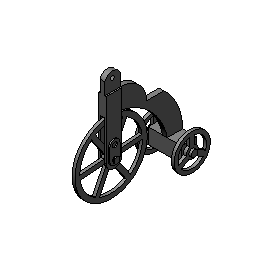
Monkey_Riding_Bike v2 (Autodesk Fusion 360 design; units mm, degrees)
Autodesk Fusion 360 part; units mm, degrees
sketch "Wheels holder" plane through (0, 0, 0) normal (1, 0, 0) x (0, 1, 0) in component "Bike"
  line L0 (89.0864, -65.3231) -> (57.0864, -65.3231)
  line L1 (57.0864, -65.3231) -> (57.0864, -97.3231)
  line L2 (57.0864, -97.3231) -> (89.0864, -97.3231)
  line L3 (89.0864, -97.3231) -> (89.0864, -65.3231)
  line L4 (89.0864, -65.3231) -> (57.0864, -97.3231) construction
  line L5 (57.0864, -65.3231) -> (89.0864, -97.3231) construction
  point P0 (73.0864, -81.3231)
  dimension "d1" = 32
  dimension "d2" = 32
  constraint horizontal L0
  constraint perpendicular L0 L1
  constraint parallel L0 L2
  constraint parallel L1 L3
  constraint coincident L4 P0
  constraint coincident L5 P0
  measures "d1" distance of L1.end L2.end
  measures "d2" distance of L0.end L1.end
extrude "Extrude1" add sketch "Wheels holder" along normal mid plane 69 makes body 1 in component "Bike"
sketch "Bike" plane through (0, 0, 0) normal (1, 0, 0) x (0, 1, 0) in component "Bike"
  line L0 (50.0158, 22.6931) -> (15, 22.6931)
  line L1 (-40, 75) -> (-40, 100)
  line L2 (-72.5145, 100) -> (-72.5145, 35)
  line L3 (57.3009, -65.5095) -> (89.0864, -65.3233)
  arc A0 (57.3009, -65.5095) -> (-72.5145, 35) centre (-65.2547, -89.7112) ccw
  arc A1 (89.0864, -65.3233) -> (50.0158, 22.6931) centre (-30.4896, -65.7234) ccw
  arc A2 (15, 22.6931) -> (-40, 75) centre (-39.9292, 20.0051) ccw
  arc A3 (-40, 100) -> (-72.5145, 100) centre (-56.2572, 94.6148) ccw
  constraint horizontal L0
  constraint vertical L1
extrude "Extrude2" add sketch "Bike" along normal mid plane 10 bodies 1 in component "Bike"
sketch "Wheel" plane through (0, 0, 0) normal (1, 0, 0) x (0, 1, 0) in component "Big wheel"
  circle A0 centre (-57.5, -44) radius 75
  line L0 (-57.6215, -58.9995) -> (-40.7303, -106.7995)
  line L1 (-48.5271, -56.0203) -> (-31.6934, -103.6575)
  line L2 (-44.5708, -51.605) -> (5.2708, -60.8767)
  line L3 (-42.6037, -42.2394) -> (7.0682, -51.4796)
  line L4 (-44.4493, -36.6055) -> (-11.4989, 1.9228)
  line L5 (-51.5765, -30.2191) -> (-18.7384, 8.1779)
  line L6 (-57.3785, -29.0005) -> (-74.2697, 18.7995)
  line L7 (-66.4729, -31.9797) -> (-83.3066, 15.6575)
  line L8 (-70.4292, -36.395) -> (-120.2708, -27.1233)
  line L9 (-72.3963, -45.7606) -> (-122.0682, -36.5204)
  line L10 (-70.5507, -51.3945) -> (-103.5011, -89.9228)
  line L11 (-63.4235, -57.7809) -> (-96.2616, -96.1779)
  arc A1 (-18.7384, 8.1779) -> (-74.2697, 18.7995) centre (-57.5, -44) ccw
  arc A2 (-51.5765, -30.2191) -> (-57.3785, -29.0005) centre (-57.5, -44) ccw
  arc A3 (-42.6037, -42.2394) -> (-44.4493, -36.6055) centre (-57.5, -44) ccw
  arc A4 (7.0682, -51.4796) -> (-11.4989, 1.9228) centre (-57.5, -44) ccw
  arc A5 (-48.5271, -56.0203) -> (-44.5708, -51.605) centre (-57.5, -44) ccw
  arc A6 (-63.4235, -57.7809) -> (-57.6215, -58.9995) centre (-57.5, -44) ccw
  arc A7 (-66.4729, -31.9797) -> (-70.4292, -36.395) centre (-57.5, -44) ccw
  arc A8 (-72.3963, -45.7606) -> (-70.5507, -51.3945) centre (-57.5, -44) ccw
  arc A9 (-83.3066, 15.6575) -> (-120.2708, -27.1233) centre (-57.5, -44) ccw
  arc A10 (-122.0682, -36.5204) -> (-103.5011, -89.9228) centre (-57.5, -44) ccw
  arc A11 (-96.2616, -96.1779) -> (-40.7303, -106.7995) centre (-57.5, -44) ccw
  arc A12 (-31.6934, -103.6575) -> (5.2708, -60.8767) centre (-57.5, -44) ccw
  dimension "d7" = 150
  dimension "d9" = 30
  dimension "d11" = 360
  constraint concentric A0 A7
  constraint coincident L0.end A9
  constraint coincident L1.start A7
  constraint coincident L1.end A9
  constraint parallel L0 L1
  constraint concentric A0 A9
  constraint concentric A1 A9
  constraint concentric A2 A7
  constraint concentric A3 A7
  constraint concentric A4 A9
  constraint concentric A5 A7
  constraint concentric A6 A7
  constraint concentric A7 A8
  constraint concentric A9 A10
  constraint concentric A10 A11
  constraint concentric A11 A12
  measures "d7" diameter of A0
  measures "d9" diameter of A7
extrude "Extrude1'" add sketch "Wheel" along normal mid plane 6 separate body makes body 2 in component "Big wheel"
sketch "Wheel (2)" plane through (0, 0, 0) normal (1, 0, 0) x (0, 1, 0) in component "Small wheels"
  circle A0 centre (73.0864, -81.3232) radius 37.5
  line L0 (68.0057, -69.9023) -> (68.0057, -52.264)
  line L1 (78.1671, -69.9023) -> (78.1671, -52.264)
  line L2 (65.7359, -91.4336) -> (50.4607, -100.2528)
  line L3 (60.6552, -82.6336) -> (45.38, -91.4528)
  line L4 (85.5175, -82.6336) -> (100.7927, -91.4528)
  line L5 (80.4368, -91.4336) -> (95.712, -100.2528)
  arc A1 (68.0057, -52.264) -> (45.38, -91.4528) centre (73.0864, -81.3232) ccw
  arc A2 (68.0057, -69.9023) -> (60.6552, -82.6336) centre (73.0864, -81.3232) ccw
  arc A3 (65.7359, -91.4336) -> (80.4368, -91.4336) centre (73.0864, -81.3232) ccw
  arc A4 (85.5175, -82.6336) -> (78.1671, -69.9023) centre (73.0864, -81.3232) ccw
  arc A5 (50.4607, -100.2528) -> (95.712, -100.2528) centre (73.0864, -81.3232) ccw
  arc A6 (100.7927, -91.4528) -> (78.1671, -52.264) centre (73.0864, -81.3232) ccw
  dimension "d14" = 75
  dimension "d16" = 25
  dimension "d18" = 360
  constraint concentric A0 A3
  constraint coincident L0.start A3
  constraint vertical L0
  constraint parallel L0 L1
  constraint concentric A0 A1
  constraint concentric A1 A5
  constraint concentric A2 A3
  constraint concentric A3 A4
  constraint concentric A5 A6
  measures "d14" diameter of A0
  measures "d16" diameter of A3
extrude "Extrude1''" add sketch "Wheel (2)" along normal blind 41 and the other way blind -35 separate body makes body 3 in component "Small wheels"
extrude "Extrude2'" add sketch "Wheel (2)" along normal blind -35 and the other way blind 41 separate body makes body 4 in component "Small wheels"
sketch "Bike pedals and wheel holder" plane through (5, 0, 0) normal (1, 0, 0) x (0, 1, 0) in component "Bike"
  line L0 (57.264, -65.3231) -> (89.0864, -65.3231)
  arc A0 (89.0864, -65.3231) -> (50.0158, 22.6931) centre (-30.4896, -65.7234) ccw
  line L1 (50.0158, 22.6931) -> (15, 22.6931)
  arc A1 (15, 22.6931) -> (-40, 75) centre (-39.9292, 20.0051) ccw
  line L2 (-40, 75) -> (-40, 100)
  arc A2 (-40, 100) -> (-72.5145, 100) centre (-56.2572, 94.6148) ccw
  line L3 (-72.5145, 100) -> (-72.5145, 35)
  arc A3 (57.264, -65.3231) -> (-72.5145, 35) centre (-65.2547, -89.7112) ccw
  line L4 (-40, 75) -> (-72.5145, 75)
  line L5 (-72.5145, 75) -> (-72.5145, -46.3572)
  line L6 (-40, -46.3572) -> (-40, 75)
  arc A4 (-72.5145, -46.3572) -> (-40, -46.3572) centre (-56.2572, -46.3572) ccw
  constraint horizontal L4
  constraint vertical L5
  constraint vertical L6
  constraint coincident A1.end L2.start
  constraint tangent L5 A4
extrude "Extrude3" add sketch "Bike pedals and wheel holder" along normal blind 3 contours A3 L5 L6 A4 | L3 A3 L4 L5 L6 bodies 1 in component "Bike"
extrude "Extrude4" add sketch "Bike pedals and wheel holder" along normal blind -10 and the other way blind 13 contours A3 L5 L6 A4 | L3 A3 L4 L5 L6 bodies 1 in component "Bike"
sketch "Bike hole" plane through (5, 0, 0) normal (1, 0, 0) x (0, 1, 0) in component "Bike"
  circle A0 centre (-56.5863, 99.3164) radius 4
  dimension "d33" = 8
  measures "d33" diameter of A0
extrude "Extrude5" cut sketch "Bike hole" against normal blind 175 bodies 1 in component "Bike"
sketch "Wheel Hole" plane through (41, 0, 0) normal (1, 0, 0) x (0, 1, 0) in component "Small wheels"
  line L0 (100.7927, -91.4528) -> (85.5175, -82.6336)
  arc A0 (85.5175, -82.6336) -> (78.1671, -69.9023) centre (73.0864, -81.3232) ccw
  line L1 (78.1671, -69.9023) -> (78.1671, -52.264)
  arc A1 (100.7927, -91.4528) -> (78.1671, -52.264) centre (73.0864, -81.3232) ccw
  arc A2 (68.0057, -52.264) -> (45.38, -91.4528) centre (73.0864, -81.3232) ccw
  line L2 (68.0057, -52.264) -> (68.0057, -69.9023)
  arc A3 (68.0057, -69.9023) -> (60.6552, -82.6336) centre (73.0864, -81.3232) ccw
  line L3 (60.6552, -82.6336) -> (45.38, -91.4528)
  line L4 (50.4607, -100.2528) -> (65.7359, -91.4336)
  arc A4 (65.7359, -91.4336) -> (80.4368, -91.4336) centre (73.0864, -81.3232) ccw
  line L5 (80.4368, -91.4336) -> (95.712, -100.2528)
  arc A5 (50.4607, -100.2528) -> (95.712, -100.2528) centre (73.0864, -81.3232) ccw
  circle A6 centre (73.0864, -81.3232) radius 37.5
  circle A7 centre (73.0864, -81.3232) radius 3.9
  circle A8 centre (73.0864, -81.3232) radius 3.5
  dimension "d36" = 7.8
  dimension "d72" = -0.4
  constraint concentric A0 A7
  measures "d36" diameter of A7
sketch "Wheel hole" plane through (3, -1, 0) normal (1, 0, 0) x (0, 1, 0) in component "Big wheel"
  line L0 (-30.6934, -103.6575) -> (-47.5271, -56.0203)
  arc A0 (-47.5271, -56.0203) -> (-43.5708, -51.605) centre (-56.5, -44) ccw
  line L1 (-43.5708, -51.605) -> (6.2708, -60.8767)
  arc A1 (-30.6934, -103.6575) -> (6.2708, -60.8767) centre (-56.5, -44) ccw
  line L2 (8.0682, -51.4796) -> (-41.6037, -42.2394)
  arc A2 (-41.6037, -42.2394) -> (-43.4493, -36.6055) centre (-56.5, -44) ccw
  line L3 (-43.4493, -36.6055) -> (-10.4989, 1.9228)
  arc A3 (8.0682, -51.4796) -> (-10.4989, 1.9228) centre (-56.5, -44) ccw
  line L4 (-82.3066, 15.6575) -> (-65.4729, -31.9797)
  arc A4 (-65.4729, -31.9797) -> (-69.4292, -36.395) centre (-56.5, -44) ccw
  line L5 (-69.4292, -36.395) -> (-119.2708, -27.1233)
  arc A5 (-82.3066, 15.6575) -> (-119.2708, -27.1233) centre (-56.5, -44) ccw
  arc A6 (-17.7384, 8.1779) -> (-73.2697, 18.7995) centre (-56.5, -44) ccw
  line L6 (-17.7384, 8.1779) -> (-50.5765, -30.2191)
  arc A7 (-50.5765, -30.2191) -> (-56.3785, -29.0005) centre (-56.5, -44) ccw
  line L7 (-56.3785, -29.0005) -> (-73.2697, 18.7995)
  line L8 (-121.0682, -36.5204) -> (-71.3963, -45.7606)
  arc A8 (-71.3963, -45.7606) -> (-69.5507, -51.3945) centre (-56.5, -44) ccw
  line L9 (-69.5507, -51.3945) -> (-102.5011, -89.9228)
  arc A9 (-121.0682, -36.5204) -> (-102.5011, -89.9228) centre (-56.5, -44) ccw
  line L10 (-95.2616, -96.1779) -> (-62.4235, -57.7809)
  arc A10 (-62.4235, -57.7809) -> (-56.6215, -58.9995) centre (-56.5, -44) ccw
  line L11 (-56.6215, -58.9995) -> (-39.7303, -106.7995)
  arc A11 (-95.2616, -96.1779) -> (-39.7303, -106.7995) centre (-56.5, -44) ccw
  circle A12 centre (-56.5, -44) radius 75
  circle A13 centre (-56.5, -44) radius 5
  dimension "d47" = 10
  constraint concentric A0 A13
  measures "d47" diameter of A13
extrude "Extrude8" cut sketch "Wheel hole" along normal mid plane 40 contours A13 bodies 1 in component "Bike"
extrude "Extrude2''" cut sketch "Wheel hole" along normal mid plane 40 contours A13 bodies 2 in component "Big wheel"
sketch "Pedal" plane through (8, 0, 0) normal (1, 0, 0) x (0, 1, 0) in component "Pedals"
  circle A0 centre (-57.5, -44) radius 5
  arc A1 (-72.5145, -46.3572) -> (-40, -46.3572) centre (-56.2572, -46.3572) ccw
  line L0 (-40, -46.3572) -> (-40, 75)
  line L1 (-40, 75) -> (-72.5145, 75)
  line L2 (-72.5145, 75) -> (-72.5145, -46.3572)
  line L3 (-47, -44) -> (-47, -18)
  arc A2 (-47, -18) -> (-68, -18) centre (-57.5, -18) ccw
  line L4 (-68, -18) -> (-68, -44)
  arc A3 (-68, -44) -> (-47, -44) centre (-57.5, -44) ccw
  line L5 (-57.5, -44) -> (-57.5, -18) construction
  circle A4 centre (-57.5, -44) radius 5
  circle A5 centre (-57.5, -18) radius 5
  dimension "d52" = 10
  constraint tangent L3 A2
  constraint tangent A2 L4
  constraint parallel L3 L4
  constraint tangent L4 A3
  constraint tangent L3 A3
  constraint vertical L5
  constraint coincident A0.centre A3.centre
  constraint concentric A3 A4
  constraint concentric A2 A5
  measures "d52" diameter of A5
extrude "Extrude1'''" add sketch "Pedal" along normal blind 3 separate body contours L3 A2 L4 A3 makes body 5 in component "Pedals"
extrude "Extrude2'''" add sketch "Pedal" along normal blind -19 and the other way blind 16 separate body contours L3 A2 L4 A3 makes body 6 in component "Pedals"
extrude "Extrude9" cut sketch "Wheel Hole" against normal blind 85 contours A7 | A8 bodies 1 in component "Bike"
move_face "OffsetFaces1" offset -0.3 1 faces at (11.5, 76.967, -81.7115) on bodies 1 in component "Bike"
extrude "Extrude3'" add sketch "Pedal" along normal blind -21 and the other way blind -5 separate body contours A0 A4 makes body 7 in component "Pedals"
move_face "OffsetFaces1'" offset -0.3 1 faces at (4.3333, -52.5248, -44.4978) on bodies 7 in component "Pedals"
move_face "OffsetFaces2" offset -0.4 2 faces at (8, -65.7218, -27.8003) (-8, -65.7218, -27.8003) on bodies 5 6 in component "Pedals"
extrude "Extrude6" cut sketch "Wheel Hole" against normal blind 160 contours A7 | A8 bodies 3 4 in component "Small wheels"
extrude "Extrude7" add sketch "Wheel Hole" along normal blind -30 and the other way blind 0 separate body contours A8 makes body 8 in component "Small wheels"
extrude "Extrude8'" add sketch "Wheel Hole" along normal blind -51 and the other way blind 82 separate body contours A8 makes body 9 in component "Small wheels"
sketch "Wheel screw" plane through (41, 0, 0) normal (1, 0, 0) x (0, 1, 0) in component "Small wheels"
  circle A0 centre (73.0864, -81.3232) radius 3.5
  circle A1 centre (73.0864, -81.3232) radius 7
  dimension "d81" = 14
  constraint concentric A0 A1
  measures "d81" diameter of A1
extrude "Extrude9'" add sketch "Wheel screw" along normal blind 5 contours A0 | A1 bodies 8 in component "Small wheels"
extrude "Extrude10" add sketch "Wheel screw" along normal blind -82 and the other way blind 87 contours A0 | A1 bodies 9 in component "Small wheels"
sketch "Connecting rod" plane through (13, 0, 0) normal (1, 0, 0) x (0, 1, 0) in component "Pedals"
  circle A0 centre (-57.5, -44) radius 4.7
  circle A1 centre (-57.5, -44) radius 6
  dimension "d88" = 12
  constraint concentric A0 A1
  measures "d88" diameter of A1
extrude "Extrude4'" add sketch "Connecting rod" along normal blind 2 contours A0 | A1 bodies 7 in component "Pedals"
component "Bike" placed x (1, 0, 0) y (0, 1, 0) z (0, 0, 1) at (0, 0, 0)
component "Big wheel" placed x (1, 0, 0) y (0, 1, 0) z (0, 0, 1) at (0, 0, 0)
component "Small wheels" placed x (1, 0, 0) y (0, 1, 0) z (0, 0, 1) at (0, 0, 0)
component "Pedals" placed x (1, 0, 0) y (0, 1, 0) z (0, 0, 1) at (0, 0, 0)
named bodies: "Bike", "Wheel", "Left wheel", "Right wheel", "Left Pedal", "Right Pedal", "Left wheel screw", "Right wheels screw", "Connecting rod"
